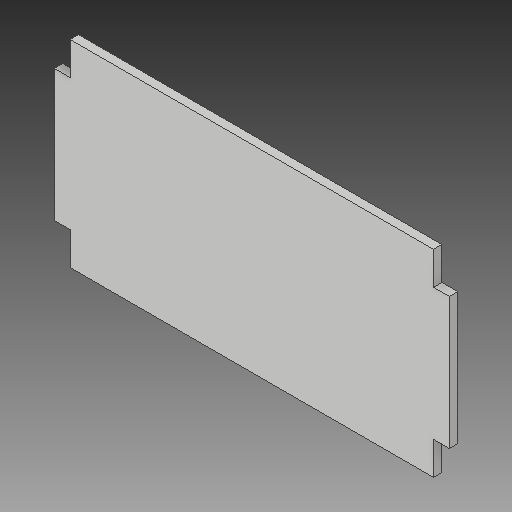
# Autodesk Inventor part: Base
Saved by Autodesk Inventor 2019 (Build 230136000, 136)
## iProperties
Created: 2020-02-10
Part Number: Base
Material: Generic
Document SubType Name: Modeling
Designer: Elías Sánchez
Density: 1 g/cm^3
Appearance: Default
Description: Corte Láser
Author: Elías Sánchez
Revision Number: IR
Autodesk Inventor part; units mm, degrees
ref_plane "YZ Plane" through (0, 0, 0) normal (1, 0, 0) x (0, 1, 0)
ref_plane "XZ Plane" through (0, 0, 0) normal (0, 1, 0) x (-1, 0, 0)
ref_plane "XY Plane" through (0, 0, 0) normal (0, 0, 1) x (1, 0, 0)
sketch "Sketch1" plane through (0, 0, 0) normal (0, 0, 1) x (1, 0, 0)
  line L0 (0, 0) -> (138, 0)
  line L1 (138, 75) -> (0, 75)
  line L2 (0, 75) -> (0, 62.5)
  line L3 (0, 62.5) -> (-6, 62.5)
  line L4 (-6, 62.5) -> (-6, 12.5)
  line L5 (-6, 12.5) -> (0, 12.5)
  line L6 (0, 12.5) -> (0, 0)
  line L7 (138, 75) -> (138, 62.5)
  line L8 (138, 62.5) -> (144, 62.5)
  line L9 (144, 62.5) -> (144, 12.5)
  line L10 (144, 12.5) -> (138, 12.5)
  line L11 (138, 12.5) -> (138, 0)
  dimension "d0" = 75
  dimension "d1" = 138
  dimension "d2" = 50
  dimension "d3" = 50
  dimension "d4" = 12.5
  dimension "d5" = 12.5
  dimension "d10" = 6
  dimension "d11" = 6
  constraints: 24 end point, 8 perpendicular, 2 point on line, 2 vertical, 1 horizontal, 1 parallel
  measures "d0" distance of L0.end L1.start
  measures "d1" distance of L1.start L1.end
  measures "d2" distance of L3.end L4.end
  measures "d3" distance of L8.end L9.end
  measures "d4" distance of L1.start L7.end
  measures "d5" distance of L1.end L2.end
  measures "d10" distance between parallel lines of L2 L4
  measures "d11" distance between parallel lines of L7 L9
extrude "Extrusion1" add sketch "Sketch1" along normal blind 3.2
equation "\"d5\" = d4"
equation "\"d11\" = d10"
body "Solid1"
